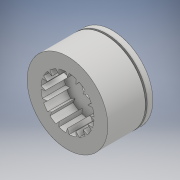
# Autodesk Inventor part: Adapter
Saved by Autodesk Inventor 2018 (Build 220112000, 112)
## iProperties
Created: 2017-12-15
Part Number: Adapter
Material: Generic
Document SubType Name: Modeling
Designer: erwin
Density: 1 g/cm^3
Appearance: Default
Author: erwin
Autodesk Inventor part; units mm, degrees
ref_plane "YZ Plane" through (0, 0, 0) normal (1, 0, 0) x (0, 1, 0)
ref_plane "XZ Plane" through (0, 0, 0) normal (0, 1, 0) x (-1, 0, 0)
ref_plane "XY Plane" through (0, 0, 0) normal (0, 0, 1) x (1, 0, 0)
sketch "Sketch1" plane through (0, 0, 0) normal (0, 1, 0) x (-1, 0, 0)
  line L0 (3.8, 0) -> (4.591, -0.2879)
  line L1 (3.8, 0) -> (5.6031, 0) construction
  line L2 (3.8, 0) -> (4.591, 0.2879)
  line L3 (3.8, 0) -> (5.3258, 0) construction
  circle A0 centre (0, 0) radius 7
  line L4 (3.5107, 1.4542) -> (4.3517, 1.4909)
  line L5 (3.5107, 1.4542) -> (5.1766, 2.1442) construction
  line L6 (3.5107, 1.4542) -> (4.1313, 2.0229)
  line L7 (3.5107, 1.4542) -> (4.9204, 2.0381) construction
  line L8 (2.687, 2.687) -> (3.4499, 3.0427)
  line L9 (2.687, 2.687) -> (3.962, 3.962) construction
  line L10 (2.687, 2.687) -> (3.0427, 3.4499)
  line L11 (2.687, 2.687) -> (3.7659, 3.7659) construction
  line L12 (1.4542, 3.5107) -> (2.0229, 4.1313)
  line L13 (1.4542, 3.5107) -> (2.1442, 5.1766) construction
  line L14 (1.4542, 3.5107) -> (1.4909, 4.3517)
  line L15 (1.4542, 3.5107) -> (2.0381, 4.9204) construction
  line L16 (0, 3.8) -> (0.2879, 4.591)
  line L17 (0, 3.8) -> (0, 5.6031) construction
  line L18 (0, 3.8) -> (-0.2879, 4.591)
  line L19 (0, 3.8) -> (0, 5.3258) construction
  line L20 (-1.4542, 3.5107) -> (-1.4909, 4.3517)
  line L21 (-1.4542, 3.5107) -> (-2.1442, 5.1766) construction
  line L22 (-1.4542, 3.5107) -> (-2.0229, 4.1313)
  line L23 (-1.4542, 3.5107) -> (-2.0381, 4.9204) construction
  line L24 (-2.687, 2.687) -> (-3.0427, 3.4499)
  line L25 (-2.687, 2.687) -> (-3.962, 3.962) construction
  line L26 (-2.687, 2.687) -> (-3.4499, 3.0427)
  line L27 (-2.687, 2.687) -> (-3.7659, 3.7659) construction
  line L28 (-3.5107, 1.4542) -> (-4.1313, 2.0229)
  line L29 (-3.5107, 1.4542) -> (-5.1766, 2.1442) construction
  line L30 (-3.5107, 1.4542) -> (-4.3517, 1.4909)
  line L31 (-3.5107, 1.4542) -> (-4.9204, 2.0381) construction
  line L32 (-3.8, 0) -> (-4.591, 0.2879)
  line L33 (-3.8, 0) -> (-5.6031, 0) construction
  line L34 (-3.8, 0) -> (-4.591, -0.2879)
  line L35 (-3.8, 0) -> (-5.3258, 0) construction
  line L36 (-3.5107, -1.4542) -> (-4.3517, -1.4909)
  line L37 (-3.5107, -1.4542) -> (-5.1766, -2.1442) construction
  line L38 (-3.5107, -1.4542) -> (-4.1313, -2.0229)
  line L39 (-3.5107, -1.4542) -> (-4.9204, -2.0381) construction
  line L40 (-2.687, -2.687) -> (-3.4499, -3.0427)
  line L41 (-2.687, -2.687) -> (-3.962, -3.962) construction
  line L42 (-2.687, -2.687) -> (-3.0427, -3.4499)
  line L43 (-2.687, -2.687) -> (-3.7659, -3.7659) construction
  line L44 (-1.4542, -3.5107) -> (-2.0229, -4.1313)
  line L45 (-1.4542, -3.5107) -> (-2.1442, -5.1766) construction
  line L46 (-1.4542, -3.5107) -> (-1.4909, -4.3517)
  line L47 (-1.4542, -3.5107) -> (-2.0381, -4.9204) construction
  line L48 (0, -3.8) -> (-0.2879, -4.591)
  line L49 (0, -3.8) -> (0, -5.6031) construction
  line L50 (0, -3.8) -> (0.2879, -4.591)
  line L51 (0, -3.8) -> (0, -5.3258) construction
  line L52 (1.4542, -3.5107) -> (1.4909, -4.3517)
  line L53 (1.4542, -3.5107) -> (2.1442, -5.1766) construction
  line L54 (1.4542, -3.5107) -> (2.0229, -4.1313)
  line L55 (1.4542, -3.5107) -> (2.0381, -4.9204) construction
  line L56 (2.687, -2.687) -> (3.0427, -3.4499)
  line L57 (2.687, -2.687) -> (3.962, -3.962) construction
  line L58 (2.687, -2.687) -> (3.4499, -3.0427)
  line L59 (2.687, -2.687) -> (3.7659, -3.7659) construction
  line L60 (3.5107, -1.4542) -> (4.1313, -2.0229)
  line L61 (3.5107, -1.4542) -> (5.1766, -2.1442) construction
  line L62 (3.5107, -1.4542) -> (4.3517, -1.4909)
  line L63 (3.5107, -1.4542) -> (4.9204, -2.0381) construction
  arc A1 (4.1313, 2.0229) -> (3.4499, 3.0427) centre (0, 0) ccw
  arc A2 (4.591, 0.2879) -> (4.3517, 1.4909) centre (0, 0) ccw
  arc A3 (4.3517, -1.4909) -> (4.591, -0.2879) centre (0, 0) ccw
  arc A4 (3.4499, -3.0427) -> (4.1313, -2.0229) centre (0, 0) ccw
  arc A5 (2.0229, -4.1313) -> (3.0427, -3.4499) centre (0, 0) ccw
  arc A6 (-4.591, -0.2879) -> (-4.3517, -1.4909) centre (0, 0) ccw
  arc A7 (-4.1313, -2.0229) -> (-3.4499, -3.0427) centre (0, 0) ccw
  arc A8 (-3.0427, -3.4499) -> (-2.0229, -4.1313) centre (0, 0) ccw
  arc A9 (-1.4909, -4.3517) -> (-0.2879, -4.591) centre (0, 0) ccw
  arc A10 (0.2879, -4.591) -> (1.4909, -4.3517) centre (0, 0) ccw
  arc A11 (3.0427, 3.4499) -> (2.0229, 4.1313) centre (0, 0) ccw
  arc A12 (1.4909, 4.3517) -> (0.2879, 4.591) centre (0, 0) ccw
  arc A13 (-0.2879, 4.591) -> (-1.4909, 4.3517) centre (0, 0) ccw
  arc A14 (-2.0229, 4.1313) -> (-3.0427, 3.4499) centre (0, 0) ccw
  arc A15 (-3.4499, 3.0427) -> (-4.1313, 2.0229) centre (0, 0) ccw
  arc A16 (-4.3517, 1.4909) -> (-4.591, 0.2879) centre (0, 0) ccw
  dimension "d2" = 20
  dimension "d3" = 20
  dimension "d7" = 360
  dimension "d38" = 14
  dimension "d39" = 4.6
  constraints: 128 end point, 32 point on circle, 17 centre point, 2 horizontal, 1 coincident, 145 other
  measures "d2" angle of L0 L1
  measures "d3" angle of L3 L2
  measures "d38" diameter of A0
  measures "d39" radius of A13
extrude "Extrusion1" add sketch "Sketch1" along normal blind 4
sketch "Sketch2" plane through (0, 4, 0) normal (0, 1, 0) x (1, 0, 0)
  circle A0 centre (0, 0) radius 7 projected
extrude "Extrusion2" add sketch "Sketch2" along normal blind 1
sketch "Sketch3" plane through (0, 5, 0) normal (0, 1, 0) x (1, 0, 0)
  arc A0 (-3.2619, 0.5) -> (-3.2619, -0.5) centre (0, 0) ccw
  line L0 (-5.9161, -1) -> (-3.2619, -0.5)
  line L1 (-5.9161, 1) -> (-3.2619, 0.5)
  line L2 (0, 0) -> (0, 6) construction
  arc A1 (3.2619, -0.5) -> (3.2619, 0.5) centre (0, 0) ccw
  line L3 (5.9161, -1) -> (3.2619, -0.5)
  line L4 (5.9161, 1) -> (3.2619, 0.5)
  arc A2 (-5.9161, -1) -> (5.9161, -1) centre (0, 0) ccw
  arc A3 (5.9161, 1) -> (-5.9161, 1) centre (0, 0) ccw
  circle A4 centre (0, 0) radius 7 projected
  point P0 (-3.3, 0)
  point P1 (3.3, 0)
  constraints: 11 point on circle, 10 end point, 5 symmetric about line, 4 centre point, 2 coincident, 1 vertical, 1 other
extrude "Extrusion3" add sketch "Sketch3" along normal blind 1.5
sketch "Sketch4" plane through (0, 5, 0) normal (0, 1, 0) x (1, 0, 0)
  point P0 (0, 0)
hole "Hole1" at (0, 5, 0) direction (0, -1, 0) diameter 3 depth 8 tip angle 118
thicken "Thicken1" operation add thickness 0.25 both sides no extend neighbours yes toward (0.185126, 0, -0.9827148) faces at (-5.0314, 5.5, -0.8333)
thicken "Thicken2" operation add thickness 0.25 both sides no extend neighbours yes toward (-0.185126, 0, 0.9827148) faces at (5.0314, 5.5, 0.8333)
sketch "Sketch5" plane through (0, 6.5, 0) normal (0, 1, 0) x (1, 0, 0)
  line L0 (-3.2147, 0.7455) -> (-5.8693, 1.2456) projected
  arc A0 (5.9161, 1) -> (-5.8693, 1.2456) centre (0, 0) ccw projected
  line L1 (5.9161, 1) -> (3.2619, 0.5) projected
  arc A1 (3.2147, -0.7455) -> (3.2619, 0.5) centre (0, 0) ccw projected
  line L2 (3.2147, -0.7455) -> (5.8693, -1.2456) projected
  arc A2 (-5.9161, -1) -> (5.8693, -1.2456) centre (0, 0) ccw projected
  line L3 (-5.9161, -1) -> (-3.2619, -0.5) projected
  arc A3 (-3.2147, 0.7455) -> (-3.2619, -0.5) centre (0, 0) ccw projected
  circle A4 centre (0, 0) radius 7 projected
  circle A5 centre (0, 0) radius 6.5
  dimension "d40" = 0.5
  constraints: 1 centre point
  measures "d40" radial gap between concentric circles of A4 A5
extrude "Extrusion4" add sketch "Sketch5" along normal blind 0.3 contours A5
sketch "Sketch6" plane through (0, 6.8, 0) normal (0, 1, 0) x (1, 0, 0)
  circle A0 centre (0, 0) radius 6.5 projected
  circle A1 centre (0, 0) radius 7 projected
  arc A2 (-5.9161, -1) -> (5.8693, -1.2456) centre (0, 0) ccw projected
  arc A3 (5.9161, 1) -> (-5.8693, 1.2456) centre (0, 0) ccw projected
  line L0 (5.9161, 1) -> (3.2619, 0.5) projected
  arc A4 (3.2147, -0.7455) -> (3.2619, 0.5) centre (0, 0) ccw projected
  line L1 (3.2147, -0.7455) -> (5.8693, -1.2456) projected
  arc A5 (-5.9161, -1) -> (5.8693, -1.2456) centre (0, 0) ccw projected
  line L2 (-5.9161, -1) -> (-3.2619, -0.5) projected
  arc A6 (-3.2147, 0.7455) -> (-3.2619, -0.5) centre (0, 0) ccw projected
  line L3 (-3.2147, 0.7455) -> (-5.8693, 1.2456) projected
  circle A7 centre (0, 0) radius 6.5 projected
extrude "Extrusion5" add sketch "Sketch6" along normal blind 1 contours A0 | A1
body "Solid1"
